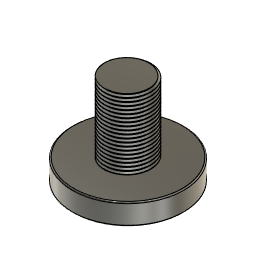
Spielteil v2 (Autodesk Fusion 360 design; units mm, degrees)
Autodesk Fusion 360 part; units mm, degrees
sketch "Skizze1" plane through (0, 0, 0) normal (0, 0, 1) x (1, 0, 0)
  circle A0 centre (0, 0) radius 47.5
  dimension "d1" = 95
  constraint coincident A0.centre origin
  measures "d1" diameter of A0
extrude "Extrusion1" add sketch "Skizze1" along normal blind 18
sketch "Skizze2" plane through (0, 0, 18) normal (0, 0, 1) x (-1, 0, 0)
  circle A0 centre (0, 0) radius 47.5
  circle A1 centre (0, 0) radius 20
  dimension "d4" = 40
  constraint coincident A0.centre A1.centre
  measures "d4" diameter of A1
extrude "Extrusion2" add sketch "Skizze2" along normal blind 60 contours A1
sketch "Skizze3" plane through (0, 0, 0) normal (0, 0, 1) x (1, 0, 0)
thread "Gewinde1" "ISO Metric profile 40.0 M40x3 6g" major diameter 39.7645 minor diameter 36.3299 pitch 3 angle 60 modelled right hand crest width 0.375 on face at (-19.9006, 1.9914, 58) crest through (-19.8822, 0, 17.8125)
fillet "Abrundung1" radius 1 2 edges at (-44.2855, -17.1767, 18) (-44.2855, -17.1767, 0)
